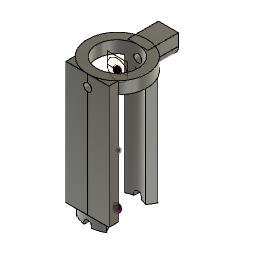
D5_To_D6 v2 (Autodesk Fusion 360 design; units mm, degrees)
Autodesk Fusion 360 part; units mm, degrees
note: some values were not read from the file. Set by a fixed rule: which sketch regions a step uses.
sketch "Main Body" plane through (0, 0, 0) normal (0, 0, 1) x (1, 0, 0)
  circle A0 centre (0, 0) radius 16.85
  circle A1 centre (0, 0) radius 24.35
  dimension "d1" = 33.7
  dimension "d2" = 48.7
  constraint coincident A0.centre A1.centre
  constraint concentric A0 A1
  measures "d1" diameter of A0
  measures "d2" diameter of A1
extrude "Extrude1" add sketch "Main Body" along normal blind 108 makes body 1
sketch "Cut Guide" plane through (0, 0, 0) normal (0, 1, 0) x (1, 0, 0)
  circle A0 centre (0, -1.28) radius 3.2
  circle A1 centre (0, -98.48) radius 3.2
  circle A2 centre (0, -98.48) radius 8.2
  line L0 (-8.2, -98.48) -> (8.2, -98.48)
  line L1 (8.2, -98.48) -> (8.2, -108)
  line L2 (8.2, -108) -> (-8.2, -108)
  line L3 (-8.2, -108) -> (-8.2, -98.48)
  point P0 (0, -41.6319)
  dimension "d5" = 6.4
  dimension "d6" = 1.28
  dimension "d11" = 6.4
  dimension "d12" = 97.2
  dimension "d13" = 16.4
  dimension "d33" = 9.52
  constraint vertical A0.centre A1.centre
  constraint vertical origin A0.centre
  constraint concentric A1 A2
  constraint horizontal L0
  constraint horizontal L2
  constraint vertical L3
  constraint coincident A2 L0.start
  constraint coincident A1.centre L0
  constraint tangent A2 L1
  constraint vertical A1.centre P0
  constraint vertical L1
  measures "d5" diameter of A0
  measures "d6" distance of origin A0.centre
  measures "d11" diameter of A1
  measures "d12" vertical distance of A0.centre A1.centre
  measures "d13" diameter of A2
  measures "d33" distance of L0.end L1.end
extrude "Extrude2" cut sketch "Cut Guide" along normal blind 24.35 and the other way blind 24.35 contours A0 bodies 1
extrude "Extrude3" add sketch "Cut Guide" along normal blind 25 from surface at 16.85 separate body contours A1 A2 L0 | A1 A2 L0 | A2 L1 L2 L3 makes body 2
sketch "Side Removal" plane through (0, 0, 0) normal (0, 0, -1) x (1, 0, 0)
  line L0 (-2.9328, 16.5928) -> (-2.9328, 24.1727)
  arc A0 (-2.9328, 24.1727) -> (-2.9328, -24.1727) centre (0, 0) ccw
  line L1 (-2.9328, -24.1727) -> (-2.9328, -16.5928)
  arc A1 (-2.9328, 16.5928) -> (-2.9328, -16.5928) centre (0, 0) ccw
  line L2 (-12.175, -21.0877) -> (12.175, 21.0877)
  arc A2 (2.9328, -24.1727) -> (2.9328, 24.1727) centre (0, 0) ccw
  line L3 (-12.175, 21.0877) -> (12.175, -21.0877)
  dimension "d19" = 120
  constraint coincident A0 L2.start
  constraint coincident L2.end A2
  constraint coincident A0 L3.start
  constraint coincident A2 L3.end
  constraint coincident L2 A0.centre
  constraint coincident L3 A0.centre
  constraint horizontal L2.end L3.start
  measures "d19" angle of L2 L3
extrude "Extrude4" cut sketch "Side Removal" against normal blind 98 contours L2 A2 L3 | A1 L2 L3 | A0 A1 L2 L3 bodies 1
sketch "Flat Bottom" plane through (0, 0, 108) normal (0, 0, 1) x (-1, 0, 0)
  circle A0 centre (0, 0) radius 16.85
  circle A1 centre (0, 0) radius 24.35
  line L0 (17.5784, 16.85) -> (-17.5784, 16.85)
  line L1 (-17.5784, 16.85) -> (-17.5784, 24.35)
  line L2 (-17.5784, 24.35) -> (17.5784, 24.35)
  line L3 (17.5784, 24.35) -> (17.5784, 16.85)
  constraint horizontal L0
  constraint vertical L1
  constraint horizontal L2
  constraint vertical L3
  constraint coincident A1 L0.start
  constraint tangent A0 L0
  constraint tangent A1 L2
  constraint coincident A1 L0.end
extrude "Extrude6" add sketch "Flat Bottom" against normal blind 100 separate body contours A1 L2 L3 | A1 L1 L2 makes body 3 at (-13.3955, -20.3343, 41.3333)
extrude "Extrude7" cut sketch "Cut Guide" along normal blind 24.35 and the other way blind 24.35 contours A1 L0 | A1 L0 bodies 1 3
equation "d2 = d1 + 15 mm"
equation "d3 = 108 mm"
equation "d6 = d5 / 5"
equation "d7 = d2 / 2"
equation "d9 = d2 / 2"
equation "d13 = d11 + 10 mm"
equation "d16 = ( d1 ) / 2"
equation "d21 = -( d3 - 10 mm )"
equation "d27 = -d3 + 8 mm"
equation "d29 = d2 / 2"
equation "d31 = d2 / 2"
equation "d33 = d3 - d12 - d6"
